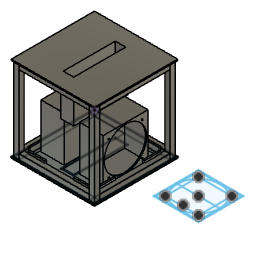
Jukebox (Autodesk Fusion 360 design; units mm, degrees)
Autodesk Fusion 360 part; units mm, degrees
sketch "Sketch1" plane through (0, 0, 0) normal (0, 0, 1) x (1, 0, 0)
  line L0 (0, 0) -> (194, 0)
  line L1 (194, 0) -> (194, -194)
  line L2 (194, -194) -> (0, -194)
  line L3 (0, -194) -> (0, 0)
  line L4 (0, -194) -> (12.5, -194)
  line L5 (12.5, -194) -> (12.5, -181.5)
  line L6 (12.5, -181.5) -> (0, -181.5)
  line L7 (0, -181.5) -> (0, -194)
  line L8 (194, 0) -> (181.5, 0)
  line L9 (181.5, 0) -> (181.5, -12.5)
  line L10 (181.5, -12.5) -> (194, -12.5)
  line L11 (194, -12.5) -> (194, 0)
  line L12 (12.5, -181.5) -> (181.5, -181.5)
  line L13 (181.5, -181.5) -> (181.5, -12.5)
  line L14 (181.5, -12.5) -> (12.5, -12.5)
  line L15 (12.5, -12.5) -> (12.5, -181.5)
  line L16 (0, 0) -> (12.5, 0)
  line L17 (12.5, 0) -> (12.5, -12.5)
  line L18 (12.5, -12.5) -> (0, -12.5)
  line L19 (0, -12.5) -> (0, 0)
  line L20 (194, -194) -> (181.5, -194)
  line L21 (181.5, -194) -> (181.5, -181.5)
  line L22 (181.5, -181.5) -> (194, -181.5)
  line L23 (194, -181.5) -> (194, -194)
  line L24 (12.5, -12.5) -> (84.5, -12.5)
  line L25 (84.5, -12.5) -> (84.5, -34.5)
  line L26 (84.5, -34.5) -> (109.5, -34.5)
  line L27 (109.5, -34.5) -> (109.5, -159.5)
  line L28 (109.5, -159.5) -> (84.5, -159.5)
  line L29 (84.5, -159.5) -> (84.5, -34.5)
  line L30 (-3, -197) -> (-3, 3)
  line L31 (-3, 3) -> (197, 3)
  line L32 (197, 3) -> (197, -197)
  line L33 (197, -197) -> (-3, -197)
  line L34 (81.5, -31.5) -> (112.5, -31.5)
  line L35 (112.5, -31.5) -> (112.5, -162.5)
  line L36 (112.5, -162.5) -> (81.5, -162.5)
  line L37 (81.5, -162.5) -> (81.5, -31.5)
  dimension "d4" = 12.5
  dimension "d108" = 25
  dimension "d109" = 125
  dimension "d157" = 194
  dimension "d160" = -3
  dimension "d161" = 37.5
  dimension "d163" = 37.5
  dimension "d164" = 87.5
  dimension "d165" = 87.5
  dimension "d170" = -3
  constraint horizontal L0
  constraint vertical L1
  constraint horizontal L2
  constraint vertical L3
  constraint coincident L0.start L3.end
  constraint horizontal L4
  constraint vertical L5
  constraint horizontal L6
  constraint vertical L7
  constraint horizontal L8
  constraint vertical L9
  constraint horizontal L10
  constraint vertical L11
  constraint equal L7 L8
  constraint equal L4 L11
  constraint equal L4 L7
  constraint horizontal L12
  constraint vertical L13
  constraint horizontal L14
  constraint vertical L15
  constraint horizontal L16
  constraint vertical L17
  constraint horizontal L18
  constraint vertical L19
  constraint horizontal L20
  constraint vertical L21
  constraint horizontal L22
  constraint vertical L23
  constraint perpendicular L15 L24
  constraint perpendicular L14 L25
  constraint horizontal L26
  constraint vertical L27
  constraint horizontal L28
  constraint vertical L29
  constraint equal L0 L3
  measures "d4" distance of L2.end L6.end
  measures "d108" distance of L25.end L26.end
  measures "d109" distance of L25.end L28.end
  measures "d157" distance of L0 L2
  measures "d161" distance of L26 L31
  measures "d163" distance of L28 L33
  measures "d164" distance of L25 L30
  measures "d165" distance of L27 L32
extrude "Extrude4" add sketch "Sketch1" along normal blind 12.5 contours L2 L5 L12 L21 makes body 1
sketch "Sketch2" plane through (12.5, 0, 0) normal (-1, 0, 0) x (0, -1, 0)
  line L0 (181.5, 0) -> (194, 0)
  line L1 (194, 0) -> (194, 12.5)
  line L2 (194, 12.5) -> (181.5, 12.5)
  line L3 (181.5, 12.5) -> (181.5, 0)
  line L4 (181.5, 0) -> (184.25, 0)
  line L5 (184.25, 0) -> (184.25, 2.75)
  line L6 (184.25, 2.75) -> (181.5, 2.75)
  line L7 (181.5, 2.75) -> (181.5, 0)
  line L8 (194, 12.5) -> (191.25, 12.5)
  line L9 (191.25, 12.5) -> (191.25, 9.75)
  line L10 (191.25, 9.75) -> (194, 9.75)
  line L11 (194, 9.75) -> (194, 12.5)
  line L12 (184.25, 2.75) -> (191.25, 2.75)
  line L13 (191.25, 2.75) -> (191.25, 9.75)
  line L14 (191.25, 9.75) -> (184.25, 9.75)
  line L15 (184.25, 9.75) -> (184.25, 2.75)
  dimension "d77" = 2.75
  dimension "d188" = 7
  constraint horizontal L4
  constraint vertical L5
  constraint horizontal L6
  constraint vertical L7
  constraint coincident L0.start L3.end
  constraint horizontal L8
  constraint vertical L9
  constraint horizontal L10
  constraint vertical L11
  constraint coincident L1.end L2.start
  constraint horizontal L12
  constraint vertical L13
  constraint horizontal L14
  constraint vertical L15
  constraint equal L4 L7
  constraint equal L7 L8
  constraint equal L7 L11
  measures "d77" distance of L0.start L6.end
  measures "d188" distance of L9.end L14.end
extrude "Extrude5" cut sketch "Sketch2" against normal blind 6 contours L12 L13 L14 L15 bodies 1
extrude "Extrude6" cut sketch "Sketch2" along normal blind 6 from surface at -169 contours L12 L13 L14 L15 bodies 1
copy_body "CopyPasteBodies1" bodies 1 makes body 2
move_body "Move1" bodies 2 to x (0, 1, 0) y (-1, 0, 0) z (0, 0, 1) at (-181.5, -194, 0)
copy_body "CopyPasteBodies2" bodies 1 makes body 3
move_body "Move2" bodies 3 to x (0, 1, 0) y (-1, 0, 0) z (0, 0, 1) at (0, -194, 0)
copy_body "CopyPasteBodies3" bodies 3 makes body 4
move_body "Move3" bodies 4 to x (0, 1, 0) y (-1, 0, 0) z (0, 0, 1) at (0, -194, 0)
copy_body "Body->Comp2" bodies 1 removing the originals makes body 5 in component "Base"
copy_body "CutPasteBodies1" bodies 2 3 4 removing the originals makes body 6 makes body 7 makes body 8 in component "Base"
extrude "Extrude1" add sketch "Sketch1" along normal blind 200 separate body contours L2 L3 L4 L5 L6 L7 makes body 9 in component "Verticals"
sketch "Sketch3" plane through (12.5, 0, 0) normal (1, 0, 0) x (0, 1, 0)
  line L0 (-194, 0) -> (-181.5, 0)
  line L1 (-181.5, 0) -> (-181.5, 200)
  line L2 (-181.5, 200) -> (-194, 200)
  line L3 (-194, 200) -> (-194, 0)
  line L4 (-194, 200) -> (-181.5, 200)
  line L5 (-181.5, 200) -> (-181.5, 187.5)
  line L6 (-181.5, 187.5) -> (-194, 187.5)
  line L7 (-194, 187.5) -> (-194, 200)
  line L8 (-184.5, 197) -> (-184.5, 190.5)
  line L9 (-184.5, 190.5) -> (-191, 190.5)
  line L10 (-191, 190.5) -> (-191, 197)
  line L11 (-191, 197) -> (-184.5, 197)
  line L12 (-194, 0) -> (-181.5, 0)
  line L13 (-181.5, 0) -> (-181.5, 12.5)
  line L14 (-181.5, 12.5) -> (-194, 12.5)
  line L15 (-194, 12.5) -> (-194, 0)
  line L16 (-184.5, 3) -> (-184.5, 9.5)
  line L17 (-184.5, 9.5) -> (-191, 9.5)
  line L18 (-191, 9.5) -> (-191, 3)
  line L19 (-191, 3) -> (-184.5, 3)
  dimension "d87" = 12.5
  dimension "d88" = 12.5
  dimension "d89" = 3
  dimension "d90" = 12.5
  dimension "d91" = 12.5
  dimension "d92" = -3
  dimension "d189" = 6.5
  constraint horizontal L4
  constraint vertical L5
  constraint horizontal L6
  constraint vertical L7
  constraint coincident L2.end L3.start
  constraint horizontal L12
  constraint vertical L13
  constraint horizontal L14
  constraint vertical L15
  constraint coincident L0.start L3.end
  measures "d87" distance of L2.end L1.end
  measures "d88" distance of L2.end L6.end
  measures "d90" distance of L0.start L0.end
  measures "d91" distance of L0.start L14.end
  measures "d189" distance of L16.end L17.end
extrude "Extrude2" add sketch "Sketch3" along normal blind 6 contours L8 L9 L10 L11 | L16 L17 L18 L19 bodies 9 in component "Verticals"
sketch "Sketch4" plane through (0, -181.5, 0) normal (0, 1, 0) x (-1, 0, 0)
  line L0 (-12.5, 0) -> (0, 0)
  line L1 (0, 0) -> (0, 200)
  line L2 (0, 200) -> (-12.5, 200)
  line L3 (-12.5, 200) -> (-12.5, 0)
  line L4 (-12.5, 200) -> (0, 200)
  line L5 (0, 200) -> (0, 187.5)
  line L6 (0, 187.5) -> (-12.5, 187.5)
  line L7 (-12.5, 187.5) -> (-12.5, 200)
  line L8 (-3, 190.5) -> (-9.5, 190.5)
  line L9 (-9.5, 190.5) -> (-9.5, 197)
  line L10 (-9.5, 197) -> (-3, 197)
  line L11 (-3, 197) -> (-3, 190.5)
  line L12 (-12.5, 0) -> (0, 0)
  line L13 (0, 0) -> (0, 12.5)
  line L14 (0, 12.5) -> (-12.5, 12.5)
  line L15 (-12.5, 12.5) -> (-12.5, 0)
  line L16 (-9.5, 3) -> (-3, 3)
  line L17 (-3, 3) -> (-3, 9.5)
  line L18 (-3, 9.5) -> (-9.5, 9.5)
  line L19 (-9.5, 9.5) -> (-9.5, 3)
  dimension "d95" = 12.5
  dimension "d96" = 12.5
  dimension "d97" = 3
  dimension "d98" = 12.5
  dimension "d99" = 12.5
  dimension "d100" = -3
  constraint horizontal L4
  constraint vertical L5
  constraint horizontal L6
  constraint vertical L7
  constraint coincident L2.end L3.start
  constraint horizontal L12
  constraint vertical L13
  constraint horizontal L14
  constraint vertical L15
  constraint coincident L0.start L3.end
  measures "d95" distance of L2.end L1.end
  measures "d96" distance of L2.end L6.end
  measures "d98" distance of L0.start L0.end
  measures "d99" distance of L0.start L14.end
extrude "Extrude3" add sketch "Sketch4" along normal blind 6 contours L8 L9 L10 L11 | L16 L17 L18 L19 bodies 9 in component "Verticals"
copy_body "CopyPasteBodies1'" bodies 9 makes body 10 in component "Verticals"
move_body "Move1'" bodies 10 to x (0, 1, 0) y (-1, 0, 0) z (0, 0, 1) at (0, -194, 0) in component "Verticals"
copy_body "CopyPasteBodies2'" bodies 10 makes body 11 in component "Verticals"
move_body "Move2'" bodies 11 to x (0, 1, 0) y (-1, 0, 0) z (0, 0, 1) at (0, -194, 0) in component "Verticals"
copy_body "CopyPasteBodies3'" bodies 9 makes body 12 in component "Verticals"
move_body "Move3'" bodies 12 to x (0, -1, 0) y (1, 0, 0) z (0, 0, 1) at (194, 0, 0) in component "Verticals"
copy_body "CopyPasteBodies4" bodies 5 makes body 13
move_body "Move4" bodies 13 to x (1, 0, 0) y (0, 1, 0) z (0, 0, 1) at (0, 0, 187.5)
copy_body "Body->Comp3" bodies 13 removing the originals makes body 14 in component "Top"
copy_body "CopyPasteBodies1''" bodies 14 makes body 15 in component "Top"
move_body "Move1''" bodies 15 to x (1, 0, 0) y (0, 1, 0) z (0, 0, 1) at (0, 181.5, 0) in component "Top"
copy_body "CopyPasteBodies2''" bodies 15 makes body 16 in component "Top"
move_body "Move2''" bodies 16 to x (0, 1, 0) y (-1, 0, 0) z (0, 0, 1) at (0, -194, 0) in component "Top"
copy_body "CopyPasteBodies3''" bodies 16 makes body 17 in component "Top"
move_body "Move3''" bodies 17 to x (1, 0, 0) y (0, 1, 0) z (0, 0, 1) at (181.5, 0, 0) in component "Top"
extrude "Extrude1'" add sketch "Sketch1" against normal blind 3 separate body contours L0 L3 L16 L17 L18 L19 | L0 L9 L14 L17 L24 | L3 L6 L15 L18 | L0 L1 L8 L9 L10 L11 | L12 L13 L14 L15 L24 | L2 L3 L4 L5 L6 L7 | L1 L10 L13 L22 | L2 L5 L12 L21 | L1 L2 L20 L21 L22 L23 | L26 L27 L28 L29 | L30 L31 L32 L33 | L34 L35 L36 L37 makes body 18 in component "Shell"
extrude "Extrude2'" add sketch "Sketch1" along normal blind 3 from surface at 200 separate body contours L0 L3 L16 L17 L18 L19 | L0 L9 L14 L17 L24 | L3 L6 L15 L18 | L0 L1 L8 L9 L10 L11 | L12 L13 L14 L15 L24 | L2 L3 L4 L5 L6 L7 | L1 L10 L13 L22 | L2 L5 L12 L21 | L1 L2 L20 L21 L22 L23 | L30 L31 L32 L33 | L34 L35 L36 L37 makes body 19 in component "Shell"
sketch "Sketch6" plane through (0, 0, 0) normal (0, 0, 1) x (1, 0, 0)
  line L0 (250, 0) -> (358, 0)
  line L1 (358, 0) -> (358, -108)
  line L2 (358, -108) -> (250, -108)
  line L3 (250, -108) -> (250, 0)
  line L4 (355, -3) -> (355, -105)
  line L5 (355, -105) -> (253, -105)
  line L6 (253, -105) -> (253, -3)
  line L7 (253, -3) -> (355, -3)
  line L8 (304, -105) -> (304, -91)
  circle A0 centre (304, -91) radius 2
  line L9 (250, -54) -> (358, -54)
  circle A1 centre (304, -54) radius 51
  line L10 (344, -14) -> (344, -94)
  line L11 (344, -94) -> (264, -94)
  line L12 (264, -94) -> (264, -14)
  line L13 (264, -14) -> (344, -14)
  circle A2 centre (264, -14) radius 2
  circle A3 centre (344, -14) radius 2
  circle A4 centre (344, -94) radius 2
  circle A5 centre (264, -94) radius 2
  dimension "d116" = 108
  dimension "d177" = 3
  dimension "d178" = 14
  dimension "d179" = 4
  dimension "d180" = 102
  dimension "d181" = 14
  dimension "d182" = 4
  constraint horizontal L0
  constraint vertical L1
  constraint horizontal L2
  constraint vertical L3
  constraint equal L0 L3
  constraint midpoint L5 L8.start
  constraint perpendicular L5 L8
  constraint coincident L8.end A0.centre
  constraint midpoint L3 L9.start
  constraint midpoint L1 L9.end
  constraint midpoint L9 A1.centre
  constraint coincident L12.end L13.start
  constraint coincident L10.start L13.end
  constraint coincident L10.end L11.start
  constraint coincident L11.end L12.start
  constraint equal A2 A3
  constraint equal A2 A4
  constraint equal A2 A5
  measures "d116" distance of L0.start L2.end
  measures "d178" distance of L8.start L8.end
  measures "d179" diameter of A0
  measures "d180" diameter of A1
  measures "d182" diameter of A2
extrude "Extrude7" add sketch "Sketch6" along normal blind 3 separate body makes body 20
copy_body "Body->Comp4" bodies 20 removing the originals makes body 21 in component "Electronics"
sketch "Sketch1 (2)" plane through (197, 0, 0) normal (1, 0, 0) x (0, 1, 0) in component "Shell"
  line L0 (-181.5, 0) -> (-12.5, 0)
  line L1 (-12.5, 0) -> (-12.5, 1)
  line L2 (-181.5, 0) -> (-181.5, 12.5)
  line L3 (-181.5, 12.5) -> (-181.5, 16)
  line L4 (-181.5, 16) -> (-177.5, 16)
  line L5 (-177.5, 16) -> (-177.5, 3)
  line L6 (-181.5, 16) -> (-183.5, 16)
  line L7 (-183.5, 16) -> (-183.5, 12.5)
  line L8 (-183.5, 12.5) -> (-181.5, 12.5)
  line L9 (-181.5, 12.5) -> (-181.5, 16)
  line L10 (-181.5, 16) -> (-183.5, 13.0681)
  line L11 (-181.5, 16) -> (-181.3024, 16) construction
  line L12 (-183.5, 13.0681) -> (-181.5, 12.5)
  line L13 (-177.5, 0) -> (-177.5, 3)
  arc A0 (-177.5, 3) -> (-174.4609, 0.0003) centre (-174.5, 3) ccw
  line L14 (3, 0) -> (-197, 0)
  line L15 (-197, 0) -> (-197, -3)
  line L16 (-197, -3) -> (3, -3)
  line L17 (3, -3) -> (3, 0)
  line L18 (-197, 0) -> (-181.5, 0)
  line L19 (-181.5, 0) -> (-177.5, 0)
  dimension "d144" = 12.5
  dimension "d145" = 3.5
  dimension "d146" = 4
  dimension "d147" = 2
  dimension "d148" = 3.5
  dimension "d149" = 124.3
  dimension "d150" = 3
  dimension "d152" = 3
  dimension "d166" = 15.5
  constraint perpendicular L3 L4
  constraint horizontal L6
  constraint vertical L7
  constraint horizontal L8
  constraint vertical L9
  constraint horizontal L11
  constraint coincident L7 L10.end
  constraint coincident L5 L13.end
  constraint coincident L13.start L5
  constraint tangent L5 A0
  constraint coincident L14.end L15.start
  constraint perpendicular L15 L18
  constraint coincident L0.start L2.start
  constraint perpendicular L4 L5
  constraint perpendicular L2 L18
  constraint collinear L3 L9
  constraint coincident L0 L13.start
  constraint parallel L0 L19
  constraint equal L4 L19
  constraint coincident L13.start L19.end
  constraint coincident L5.end L13.end
  measures "d144" distance of L0.start L2.end
  measures "d145" distance of L2.end L3.end
  measures "d146" distance of L3.end L4.end
  measures "d147" distance of L3.end L6.end
  measures "d148" distance of L3.end L2.end
  measures "d149" angle of L10 L11
  measures "d150" distance of L13.start L5.end
  measures "d152" radius of A0
  measures "d166" distance of L14.end L0.start
extrude "Extrude5'" add sketch "Sketch1 (2)" along normal blind 40 from surface at -65.5 separate body contours L0 L2 L3 L4 L5 L9 L13 L14 L19 | L0 L13 A0 L14 | L3 L9 L10 L12 makes body 22 in component "Shell"
copy_body "CopyPasteBodies3'''" bodies 22 makes body 23 in component "Shell"
move_body "Move1'''" bodies 23 to x (1, 0, 0) y (0, 1, 0) z (0, 0, 1) at (-109, 0, 0) in component "Shell"
copy_body "CopyPasteBodies4'" bodies 22 makes body 24 in component "Shell"
move_body "Move2'''" bodies 24 to x (0, 1, 0) y (-1, 0, 0) z (0, 0, 1) at (0, -303, 0) in component "Shell"
copy_body "CopyPasteBodies5" bodies 24 makes body 25 in component "Shell"
move_body "Move3'''" bodies 25 to x (1, 0, 0) y (0, 1, 0) z (0, 0, 1) at (0, 109, 0) in component "Shell"
copy_body "CopyPasteBodies6" bodies 22 makes body 26 in component "Shell"
move_body "Move4'" bodies 26 to x (-1, 0, 0) y (0, -1, 0) z (0, 0, 1) at (303, -194, 0) in component "Shell"
copy_body "CopyPasteBodies7" bodies 26 makes body 27 in component "Shell"
move_body "Move5" bodies 27 to x (1, 0, 0) y (0, 1, 0) z (0, 0, 1) at (-109, 0, 0) in component "Shell"
copy_body "CopyPasteBodies8" bodies 25 24 makes body 28 makes body 29 in component "Shell"
move_body "Move6" bodies 28 29 to x (-1, 0, 0) y (0, -1, 0) z (0, 0, 1) at (194, -194, 0) in component "Shell"
extrude "Extrude6'" add sketch "Sketch1" along normal blind 3 from surface at 197 contours L12 L13 L14 L15 L24 | L34 L35 L36 L37 bodies 19 in component "Shell"
extrude "Extrude7'" add sketch "Sketch1" against normal blind 90 from surface at 197 contours L34 L35 L36 L37 bodies 19 in component "Shell"
extrude "Extrude8" add sketch "Sketch1" against normal blind 3 from surface at 107 contours L26 L27 L28 L29 | L34 L35 L36 L37 bodies 19 in component "Shell"
extrude "Extrude1''" add sketch "Sketch6" along normal blind 56 contours L0 L1 L3 L4 L6 L7 L9 | L1 L2 L3 L4 L5 L6 L9 bodies 21 in component "Electronics"
extrude "Extrude2''" add sketch "Sketch6" along normal blind 3 from surface at 53 contours L5 L6 A1 L11 L12 A5 | L6 L7 A1 L12 L13 A2 | L4 L7 A1 L10 L13 A3 | L4 L5 A1 L10 L11 A4 | A1 L12 L13 A2 | A1 L11 L12 A5 | A1 L10 L13 A3 | A1 L10 L11 A4 bodies 21 in component "Electronics"
move_body "Move1''''" bodies 21 to x (1, 0, 0) y (0, 1, 0) z (0, 0, 1) at (0, 0, -10) in component "Electronics"
copy_body "CopyPasteBodies1'''" bodies 21 makes body 30 in component "Electronics"
move_body "Move2''''" bodies 30 to x (0, 1, 0) y (1, 0, 0) z (0, 0, -1) at (358, -358, -57) in component "Electronics"
move_body "Move3''''" bodies 21 to x (0, -1, 0) y (1, 0, 0) z (0, 0, 1) at (358, 250, 0) in component "Electronics"
component "Base" placed x (1, 0, 0) y (0, 1, 0) z (0, 0, 1) at (0, 0, 0)
component "Verticals" placed x (1, 0, 0) y (0, 1, 0) z (0, 0, 1) at (0, 0, 0)
component "Shell" placed x (1, 0, 0) y (0, 1, 0) z (0, 0, 1) at (0, 0, 0)
component "Top" placed x (1, 0, 0) y (0, 1, 0) z (0, 0, 1) at (0, 0, 0)
component "Electronics" placed x (0, 0, 1) y (0, 1, 0) z (-1, 0, 0) at (68.4612, -43, -250.0388)
named bodies: "Female Rod 0", "Female Rod", "Female Rod 1", "Female Rod (1)", "Female Rod 2", "Female Rod 3", "Female Rod 4", "Male Rod 1", "Male Rod 2", "Male Rod 3", "Male Rod 1 (1)", "Male Rod 4", "Female Rod 0 (1)", "Base", "Top", "Speaker 1", "Clip 1", "Clip 2", "Clip", "Clip 3", "Clip (1)", "Clip 4", "Clip (2)", "Clip 5", "Clip (2) (1)", "Clip 6", "Clip (1) (1)", "Clip (1) (2)", "Clip 7", "Clip 8", "Speaker 2"
